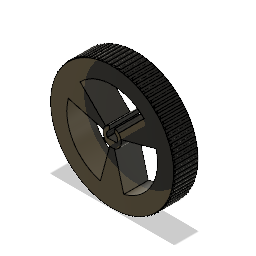
61f058dd-6cd1-40da-bcea-542ea612e3cd (Autodesk Fusion 360 design; units mm, degrees)
Autodesk Fusion 360 part; units mm, degrees
sketch "Sketch1" plane through (0, 0, 0) normal (0, 1, 0) x (1, 0, 0)
  circle A0 centre (0, 0) radius 16.75
  circle A1 centre (0, 0) radius 14.3
  line L0 (0, 0) -> (2.5, 0) construction
  line L1 (0.647048, 2.414815) -> (3.183474, 11.880888)
  line L2 (0, 0) -> (12.3, 0) construction
  line L3 (0, 0) -> (12.3, 0) construction
  line L4 (0, 0) -> (12.3, 0) construction
  line L5 (2.414815, -0.647048) -> (11.880888, -3.183474)
  line L6 (-2.414815, -0.647048) -> (-11.880888, -3.183474)
  line L7 (0, 0) -> (12.3, 0) construction
  line L8 (1.767767, -1.767767) -> (8.697413, -8.697413)
  line L9 (0, 0) -> (12.3, 0) construction
  line L10 (-1.767767, -1.767767) -> (-8.697413, -8.697413)
  line L11 (0, 0) -> (12.3, 0) construction
  line L12 (-0.647048, 2.414815) -> (-3.183474, 11.880888)
  line L13 (0, 0) -> (12.3, 0) construction
  line L14 (0, 0) -> (0, 1.5)
  arc A2 (-0.647048, 2.414815) -> (-2.414815, -0.647048) centre (0, 0) ccw
  arc A3 (2.414815, -0.647048) -> (0.647048, 2.414815) centre (0, 0) ccw
  line L15 (0, 0) -> (1.5, 0) construction
  line L16 (-0.75, -1.299038) -> (-0.75, -2.384848)
  line L17 (0.75, -1.299038) -> (0.75, -2.384848)
  line L18 (-1.307652, 0.734879) -> (1.307652, 0.734879)
  arc A4 (0.75, -2.384848) -> (-0.75, -2.384848) centre (0, 0) ccw
  arc A5 (-1.767767, -1.767767) -> (-0.75, -2.384848) centre (0, 0) ccw
  arc A6 (0.75, -2.384848) -> (1.767767, -1.767767) centre (0, 0) ccw
  arc A7 (0.75, -1.299038) -> (1.307652, 0.734879) centre (0, 0) ccw
  arc A8 (-1.307652, 0.734879) -> (-0.75, -1.299038) centre (0, 0) ccw
  arc A9 (11.880888, -3.183474) -> (3.183474, 11.880888) centre (0, 0) ccw
  arc A10 (-3.183474, 11.880888) -> (-11.880888, -3.183474) centre (0, 0) ccw
  arc A11 (-8.697413, -8.697413) -> (8.697413, -8.697413) centre (0, 0) ccw
  constraint coincident A0.centre A1.centre
  constraint coincident L0.end A2
extrude "Extrude2" add sketch "Sketch1" along normal blind 6.7 contours A1 picked at (7.581122, -4.376963) makes body 1
extrude "Extrude1" add sketch "Sketch1" along normal blind 8.65 separate body contours A2 A3 L16 L17 L18 A4 A5 A6 A7 A8 picked at (0.763926, 1.255969) makes body 2
extrude "Extrude3" add sketch "Sketch1" along normal blind 6.65 contours A0 picked at (15.817732, -1.542587) bodies 1
sketch "Sketch2" plane through (0, 6.65, 0) normal (0, 1, 0) x (-1, 0, 0)
  circle A0 centre (0, 0) radius 14.3
  circle A1 centre (0, 0) radius 16.75
  circle A2 centre (-16.74982, 0.077621) radius 0.25
  dimension "d44" = 0.5
  measures "d44" diameter of A2
extrude "Extrude4" add sketch "Sketch2" against normal blind 6.65 contours A1 A2 picked at (-16.833014, 0.078007) bodies 1
fillet "Fillet1" radius 0.25 1 edges at (16.999817, 6.65, 0.07878) on bodies 1
fillet "Fillet2" radius 0.25 1 edges at (16.999817, 0, 0.07878) on bodies 1
pattern_circular "C-Pattern1" count 90 over 360 about axis through (0, 1.75, 0) along (0, 1, 0) of 3 faces at (16.998643, 0.225704, 0.078774) (16.772993, 4.350033, -0.171303) (16.998643, 6.424296, 0.078774) on bodies 1
move_body "Move1" bodies 1 2 to x (1, 0, 0) y (0, 0, -1) z (0, 1, 0) at (-1.742373, 5.95413, -16.993848)
combine "Combine1" operation add target body 1 tool bodies 2 keep tools
